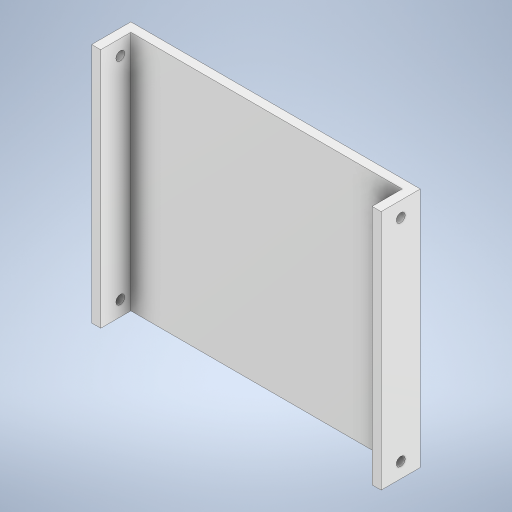
# Autodesk Inventor part: Mirror_shell_adapter
Saved by Autodesk Inventor 2023 (Build 270158000, 158)
## iProperties
Created: 2023-04-06
Part Number: Mirror_shell_adapter
Material: Generic
Document SubType Name: Modeling
Designer: ASARe-DAQ-PC
Density: 1 g/cm^3
Appearance: Default
Author: ASARe-DAQ-PC
Autodesk Inventor part; units mm, degrees
ref_plane "YZ Plane" through (0, 0, 0) normal (1, 0, 0) x (0, 1, 0)
ref_plane "XZ Plane" through (0, 0, 0) normal (0, 1, 0) x (-1, 0, 0)
ref_plane "XY Plane" through (0, 0, 0) normal (0, 0, 1) x (1, 0, 0)
sketch "Sketch1" plane through (0, 0, 0) normal (0, 0, 1) x (1, 0, 0)
  line L0 (0, 0) -> (96, 0)
  line L1 (96, 0) -> (96, 80)
  line L2 (96, 80) -> (0, 80)
  line L3 (0, 80) -> (0, 0)
  dimension "d0" = 96
  dimension "d1" = 80
  constraints: 8 end point, 2 parallel, 1 horizontal, 1 perpendicular
  measures "d0" distance of L1.end L2.end
  measures "d1" distance of L0.end L1.end
extrude "Extrusion1" add sketch "Sketch1" along normal blind 13
sketch "Sketch2" plane through (0, 80, 0) normal (0, 1, 0) x (1, 0, 0)
  line L0 (3, -13) -> (93, -13)
  line L1 (93, -13) -> (93, -3)
  line L2 (93, -3) -> (3, -3)
  line L3 (3, -3) -> (3, -13)
  line L4 (0, 0) -> (0, -13) projected
  line L5 (96, 0) -> (0, 0) projected
  line L6 (96, 0) -> (96, -13) projected
  dimension "d4" = 3
  dimension "d5" = 3
  dimension "d6" = 3
  constraints: 8 end point, 2 parallel, 1 horizontal, 1 perpendicular, 1 point on line
  measures "d4" distance between parallel lines of L4 L3
  measures "d5" distance between parallel lines of L5 L2
  measures "d6" distance between parallel lines of L6 L1
extrude "Extrusion2" cut sketch "Sketch2" against normal through all
sketch "Sketch3" plane through (96, 0, 0) normal (1, 0, 0) x (0, 0, -1)
  line L0 (0, 80) -> (-13, 80) construction
  line L1 (-6.5, 80) -> (-6.5, 0) construction
  line L2 (0, 0) -> (-13, 0) construction
  line L3 (-13, 0) -> (-13, 80) construction
  line L4 (0, 0) -> (0, 80) projected
  point P0 (-6.5, 75)
  point P1 (-6.5, 5)
  dimension "d17" = 70
  dimension "d18" = 5
  dimension "d19" = 6.5
  constraints: 2 end point, 2 midpoint, 2 point on line, 1 vertical
  measures "d17" distance of point (-6.5, 5) point (-6.5, 75)
  measures "d18" distance from line of L0 point (-6.5, 75)
  measures "d19" distance between parallel lines of L4 L1
hole "Hole1" at (96, 75, 6.5) at (96, 5, 6.5) direction (-1, 0, 0) diameter 3 end through all
body "Solid1"
